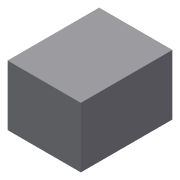
# Autodesk Inventor part: Body
Saved by Autodesk Inventor 2019 (Build 230136000, 136)
## iProperties
Created: 2019-04-28
Part Number: Body
Material: 일반
Document SubType Name: Modeling
Designer: hinmo
Density: 1 g/cm^3
Appearance: 기본값
Author: hinmo
Autodesk Inventor part; units mm, degrees
ref_plane "YZ Plane" through (0, 0, 0) normal (1, 0, 0) x (0, 1, 0)
ref_plane "XZ Plane" through (0, 0, 0) normal (0, 1, 0) x (-1, 0, 0)
ref_plane "XY Plane" through (0, 0, 0) normal (0, 0, 1) x (1, 0, 0)
sketch "스케치1" plane through (0, 0, 0) normal (1, 0, 0) x (0, 1, 0)
  line L0 (-230, 350) -> (230, 350)
  line L1 (230, 350) -> (230, -350)
  line L2 (230, -350) -> (-230, -350)
  line L3 (-230, -350) -> (-230, 350)
  line L4 (-230, 350) -> (230, -350) construction
  line L5 (230, 350) -> (-230, -350) construction
  point P0 (0, 0)
  dimension "d0" = 460
  dimension "d1" = 700
  constraints: 12 end point, 2 midpoint, 2 parallel, 1 horizontal, 1 perpendicular
  measures "d0" distance of L1.end L2.end
  measures "d1" distance of L0.end L1.end
extrude "돌출1" add sketch "스케치1" along normal blind 560
